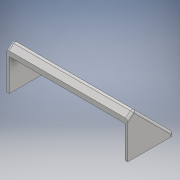
# Autodesk Inventor part: holder-LCD-screen
Saved by Autodesk Inventor 2018 (Build 220112000, 112)
## iProperties
Created: 2017-11-05
Part Number: holder-LCD-screen
Material: Generic
Document SubType Name: Modeling
Designer: Jurjen
Density: 1 g/cm^3
Appearance: Default
Author: Jurjen
Autodesk Inventor part; units mm, degrees
ref_plane "YZ Plane" through (0, 0, 0) normal (1, 0, 0) x (0, 1, 0)
ref_plane "XZ Plane" through (0, 0, 0) normal (0, 1, 0) x (-1, 0, 0)
ref_plane "XY Plane" through (0, 0, 0) normal (0, 0, 1) x (1, 0, 0)
sketch "Sketch1" plane through (0, 0, 0) normal (1, 0, 0) x (0, 1, 0)
  line L0 (-30, 24.2931) -> (-30, -24.2931)
  line L1 (30, -20.2931) -> (-21.6188, 31.3257)
  line L2 (-21.6188, 31.3257) -> (-30, 24.2931)
  line L3 (30, -20.2931) -> (30, -24.2931)
  line L4 (30, -24.2931) -> (-30, -24.2931)
  point P0 (0, 0)
  point P1 (-30, 0)
  point P2 (0, -24.2931)
  point P3 (-30, 0)
  dimension "d3" = 50
  dimension "d4" = 73
  dimension "d8" = 60
  dimension "d9" = 45
  dimension "d10" = 4
  constraints: 10 end point, 3 midpoint, 2 horizontal alignment, 2 vertical, 1 perpendicular, 1 vertical alignment
  measures "d3" angle of L2 L0
  measures "d4" distance of L1.start L1.end
  measures "d8" distance of L3.end L0.end
  measures "d9" angle of L4 L1
  measures "d10" distance of L1.start L3.end
extrude "Extrusion1" add sketch "Sketch1" along normal mid plane 160
sketch "Sketch2" plane through (-80, -21.6188, 31.3257) normal (0, 0.7071068, 0.7071068) x (1, 0, 0)
  line L0 (3.5, 69.5) -> (156.5, 69.5)
  line L1 (156.5, 69.5) -> (156.5, 3.5)
  line L2 (156.5, 3.5) -> (3.5, 3.5)
  line L3 (3.5, 3.5) -> (3.5, 69.5)
  line L4 (0, 0) -> (0, 73) projected
  line L5 (0, 0) -> (160, 0) projected
  line L6 (0, 73) -> (160, 73) projected
  line L7 (160, 73) -> (160, 0) projected
  point P0 (80, 37.4374)
  dimension "d11" = 3.5
  dimension "d12" = 3.5
  dimension "d13" = 3.5
  dimension "d14" = 3.5
  constraints: 8 end point, 2 parallel, 1 horizontal, 1 perpendicular
  measures "d11" distance between parallel lines of L4 L3
  measures "d12" distance between parallel lines of L5 L2
  measures "d13" distance between parallel lines of L6 L0
  measures "d14" distance between parallel lines of L7 L1
extrude "Extrusion2" cut sketch "Sketch2" against normal up to next contours L0 L1 L2 L3
sketch "Sketch3" plane through (-80, -21.6188, 31.3257) normal (0, 0.7071068, 0.7071068) x (1, 0, 0)
  line L0 (3.5, 3.5) -> (3.5, 69.5) projected
  line L1 (3.5, 69.5) -> (156.5, 69.5) projected
  line L2 (156.5, 69.5) -> (156.5, 3.5) projected
  line L3 (156.5, 3.5) -> (3.5, 3.5) projected
  line L4 (0, 0) -> (160, 0) projected
  line L5 (160, 73) -> (160, 0) projected
  line L6 (0, 73) -> (160, 73) projected
  line L7 (0, 0) -> (0, 73) projected
  line L8 (3.5, 69.5) -> (156.5, 69.5)
  line L9 (156.5, 69.5) -> (156.5, 3.5)
  line L10 (156.5, 3.5) -> (3.5, 3.5)
  line L11 (3.5, 3.5) -> (3.5, 69.5)
  line L12 (17.2, 55) -> (115.2, 55)
  line L13 (115.2, 55) -> (115.2, 14.5)
  line L14 (115.2, 14.5) -> (17.2, 14.5)
  line L15 (17.2, 14.5) -> (17.2, 55)
  circle A0 centre (141.6, 38.45) radius 2.25
  arc A1 (142.6, 56.45) -> (140.6, 56.45) centre (141.6, 56.45) ccw
  arc A2 (140.6, 52.45) -> (142.6, 52.45) centre (141.6, 52.45) ccw
  arc A3 (139.6, 54.95) -> (137.6, 54.95) centre (138.6, 54.95) ccw
  line L16 (140.6, 52.45) -> (140.6, 56.45)
  line L17 (142.6, 56.45) -> (142.6, 52.45)
  arc A4 (137.6, 53.95) -> (139.6, 53.95) centre (138.6, 53.95) ccw
  line L18 (137.6, 53.95) -> (137.6, 54.95)
  line L19 (139.6, 54.95) -> (139.6, 53.95)
  line L20 (141.6, 52.45) -> (141.6, 56.45) construction
  arc A5 (145.6, 54.95) -> (143.6, 54.95) centre (144.6, 54.95) ccw
  arc A6 (143.6, 53.95) -> (145.6, 53.95) centre (144.6, 53.95) ccw
  line L21 (145.6, 53.95) -> (145.6, 54.95)
  line L22 (143.6, 54.95) -> (143.6, 53.95)
  point P0 (80, 37.4374)
  dimension "d17" = 98
  dimension "d18" = 40.5
  dimension "d19" = 26.4
  dimension "d20" = 4.5
  dimension "d21" = 23.95
  dimension "d22" = 13.7
  dimension "d23" = 11
  dimension "d24" = 2
  dimension "d25" = 4
  dimension "d26" = 3
  dimension "d27" = 1.5
  dimension "d28" = 1.5
  dimension "d29" = 14
  constraints: 30 end point, 14 point on circle, 7 centre point, 7 symmetric about line, 6 tangent, 5 parallel, 3 equal radius, 3 vertical alignment, 2 horizontal, 2 perpendicular, 2 point on line, 2 vertical, 2 other
  measures "d17" distance between parallel lines of L13 L15
  measures "d18" distance between parallel lines of L14 L12
  measures "d19" distance from line of L13 A0.centre
  measures "d20" diameter of A0
  measures "d21" distance from line of A0.centre L14
  measures "d22" distance between parallel lines of L0 L15
  measures "d23" distance between parallel lines of L3 L14
  measures "d24" diameter of A1
  measures "d25" distance of L17.end L17.start
  measures "d26" horizontal distance of L20.end A3.centre
  measures "d27" vertical distance of L20.end A3.centre
  measures "d28" vertical distance of A4.centre L20.start
  measures "d29" distance of A0.centre L20.start
extrude "Extrusion3" add sketch "Sketch3" against normal blind 3 contours L0 L1 L2 L3
fillet "Fillet1" radius 3 8 edges at (0, -21.6188, 31.3257) (-80, 4.1906, 5.5163) (-80, -25.8094, 27.8094) (80, -25.8094, 27.8094) (80, 4.1906, 5.5163) (0, 30, -20.2931) (-80, 30, -22.2931) (80, 30, -22.2931)
equation "\"d12\" = d11"
equation "\"d13\" = d11"
equation "\"d14\" = d11"
equation "\"d28\" = d27"
body "Solid1"
